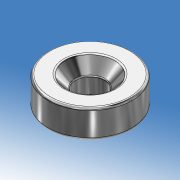
# Autodesk Inventor part: 5862K12
Saved by Autodesk Inventor 2015 SP1 (Build 190203100, 203)
## iProperties
Created: 2015-04-18
Material: STEEL, HIGH CARBON (1075/1080/1090/1095)
Vendor: MCMASTER
Document SubType Name: Modeling
Designer: JORDANJ
Mass: 1.47097 g
Surface Area: 2.40976 cm^2
Volume: 0.187385 cm^3
Density: 7.85 g/cm^3
Appearance: Chrome - Polished
Part Number: 5862K12
Description: NEODYMIUM DISC MAGNET, 3/8" DIAMETER, WITH COUNTERSUNK HOLE FOR NUMBER 4 SCREW SIZE
Project: P-171601
RuleStatus: InUse
AfterDocSave0: file://Part Number Cleaner
LAB/DEPT: STERN (LAB)
REQUESTING SCIENTIST: STERN, DAVID
SURFACE ROUGHNESS: N/A
DESIGN DEPARTMENT: HHMI: JRC - ID&F
SPECIAL FINISH: N/A
ALTERED ITEM PART NUMBER: N/A
ALTERED ITEM VENDOR: N/A
ALTERED ITEM DESCRIPTION: N/A
Revision Number: 0
Autodesk Inventor part; units mm, degrees
ref_plane "YZ Plane" through (0, 0, 0) normal (1, 0, 0) x (0, 1, 0)
ref_plane "XZ Plane" through (0, 0, 0) normal (0, 1, 0) x (-1, 0, 0)
ref_plane "XY Plane" through (0, 0, 0) normal (0, 0, 1) x (1, 0, 0)
sketch "Sketch1" plane through (0, 0, 0) normal (0, 0, 1) x (1, 0, 0)
  line L0 (1.651, 1.714) -> (1.651, 0)
  line L1 (1.651, 0) -> (4.7625, 0)
  line L2 (4.7625, 0) -> (4.7625, 3.175)
  line L3 (4.7625, 3.175) -> (2.921, 3.175)
  line L4 (2.921, 3.175) -> (1.651, 1.714)
  line L5 (0, -0.635) -> (0, 3.81) construction
  point P0 (0, 0)
  dimension "d0" = 41
  dimension "d1" = 3.302
  dimension "d2" = 9.525
  dimension "d3" = 3.175
  dimension "d4" = 5.842
  constraints: 10 end point, 2 horizontal, 2 vertical, 1 horizontal alignment
  measures "d0" angle of L4 L5
  measures "d1" diameter of L0 L5
  measures "d2" diameter of L2 L5
  measures "d3" distance of L1.end L2.end
  measures "d4" diameter of L3.end L5
revolve "Revolution1" add sketch "Sketch1" angle 360 about axis through (0, -10, 0) along (0, 1, 0)
fillet "Fillet1" radius 0.254 5 edges at (-4.7625, 3.175, 0) (-4.7625, 0, 0) (-2.921, 3.175, 0) (-1.651, 1.714, 0) (-1.651, 0, 0)
body "Solid1"
